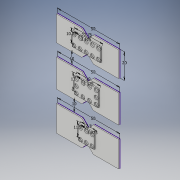
# Autodesk Inventor part: Templates
Saved by Autodesk Inventor 2017 (Build 210142000, 142)
## iProperties
Created: 2023-07-15
Part Number: Templates
Material: Generic
Document SubType Name: Modeling
Designer: Win240
Density: 1 g/cm^3
Appearance: Default
Author: Win240
Autodesk Inventor part; units mm, degrees
ref_plane "YZ Plane" through (0, 0, 0) normal (1, 0, 0) x (0, 1, 0)
ref_plane "XZ Plane" through (0, 0, 0) normal (0, 1, 0) x (-1, 0, 0)
ref_plane "XY Plane" through (0, 0, 0) normal (0, 0, 1) x (1, 0, 0)
sketch "Sketch1" plane through (0, 0, 0) normal (0, 0, 1) x (1, 0, 0)
  line L0 (-25, -11.125) -> (-4.625, -11.125)
  line L1 (25, -11.125) -> (25, 11.125)
  line L2 (25, 11.125) -> (4.625, 11.125)
  line L3 (-25, 11.125) -> (-25, -11.125)
  line L4 (-25, -11.125) -> (25, 11.125) construction
  line L5 (25, -11.125) -> (-25, 11.125) construction
  line L6 (-9.5, -6.5) -> (9.5, -6.5)
  line L7 (9.5, -6.5) -> (9.5, 6.5)
  line L8 (9.5, 6.5) -> (-9.5, 6.5)
  line L9 (-9.5, 6.5) -> (-9.5, -6.5)
  line L10 (-9.5, -6.5) -> (9.5, 6.5) construction
  line L11 (9.5, -6.5) -> (-9.5, 6.5) construction
  line L12 (0, 6.5) -> (-4.625, 11.125)
  line L13 (0, 6.5) -> (4.625, 11.125)
  line L14 (0, -6.5) -> (-4.625, -11.125)
  line L15 (0, -6.5) -> (4.625, -11.125)
  line L16 (-4.625, 11.125) -> (-25, 11.125)
  line L17 (4.625, -11.125) -> (25, -11.125)
  circle A0 centre (-7.9125, 4.9125) radius 1.5875
  circle A1 centre (-7.9125, -4.9125) radius 1.5875
  circle A2 centre (7.9125, -4.9125) radius 1.5875
  circle A3 centre (7.9125, 4.9125) radius 1.5875
  circle A4 centre (-2.6375, -4.9125) radius 1.5875
  circle A5 centre (2.6375, -4.9125) radius 1.5875
  circle A6 centre (2.6375, 4.9125) radius 1.5875
  circle A7 centre (-2.6375, 4.9125) radius 1.5875
  line L18 (-7.9125, 4.9125) -> (-2.6375, 4.9125) construction
  line L19 (2.6375, -4.9125) -> (2.6375, 4.9125) construction
  line L20 (-2.6375, 4.9125) -> (-2.6375, -4.9125) construction
  line L21 (-25, -41.675) -> (-4.625, -41.675)
  line L22 (25, -41.675) -> (25, -21.125)
  line L23 (25, -21.125) -> (4.625, -21.125)
  line L24 (-25, -21.125) -> (-25, -41.675)
  line L25 (-25, -41.675) -> (25, -21.125) construction
  line L26 (25, -41.675) -> (-25, -21.125) construction
  line L27 (-6.25, -37.05) -> (6.25, -37.05)
  line L28 (6.25, -37.05) -> (6.25, -25.75)
  line L29 (6.25, -25.75) -> (-6.25, -25.75)
  line L30 (-6.25, -25.75) -> (-6.25, -37.05)
  line L31 (-6.25, -37.05) -> (6.25, -25.75) construction
  line L32 (6.25, -37.05) -> (-6.25, -25.75) construction
  line L33 (0, -25.75) -> (-4.625, -21.125)
  line L34 (0, -25.75) -> (4.625, -21.125)
  line L35 (0, -37.05) -> (-4.625, -41.675)
  line L36 (0, -37.05) -> (4.625, -41.675)
  line L37 (-4.625, -21.125) -> (-25, -21.125)
  line L38 (4.625, -41.675) -> (25, -41.675)
  circle A8 centre (-4.6625, -27.3375) radius 1.5875
  circle A9 centre (-4.6625, -35.4625) radius 1.5875
  circle A10 centre (4.6625, -35.4625) radius 1.5875
  circle A11 centre (4.6625, -27.3375) radius 1.5875
  circle A12 centre (0, -27.3375) radius 1.5875
  circle A13 centre (0, -35.4625) radius 1.5875
  line L39 (-25, 21.125) -> (-4.625, 21.125)
  line L40 (25, 21.125) -> (25, 41.125)
  line L41 (25, 41.125) -> (4.625, 41.125)
  line L42 (-25, 41.125) -> (-25, 21.125)
  line L43 (-25, 21.125) -> (25, 41.125) construction
  line L44 (25, 21.125) -> (-25, 41.125) construction
  line L45 (-11.375, 25.75) -> (11.375, 25.75)
  line L46 (11.375, 25.75) -> (11.375, 36.5)
  line L47 (11.375, 36.5) -> (-11.375, 36.5)
  line L48 (-11.375, 36.5) -> (-11.375, 25.75)
  line L49 (-11.375, 25.75) -> (11.375, 36.5) construction
  line L50 (11.375, 25.75) -> (-11.375, 36.5) construction
  line L51 (0, 36.5) -> (-4.625, 41.125)
  line L52 (0, 36.5) -> (4.625, 41.125)
  line L53 (0, 25.75) -> (-4.625, 21.125)
  line L54 (0, 25.75) -> (4.625, 21.125)
  line L55 (-4.625, 41.125) -> (-25, 41.125)
  line L56 (4.625, 21.125) -> (25, 21.125)
  circle A14 centre (-9.7875, 34.9125) radius 1.5875
  circle A15 centre (-9.7875, 27.3375) radius 1.5875
  circle A16 centre (9.7875, 27.3375) radius 1.5875
  circle A17 centre (9.7875, 34.9125) radius 1.5875
  circle A18 centre (0, 34.9125) radius 1.5875
  circle A19 centre (0, 27.3375) radius 1.5875
  circle A20 centre (-4.8937, 27.3375) radius 1.5875
  circle A21 centre (4.8938, 27.3375) radius 1.5875
  circle A22 centre (4.8938, 34.9125) radius 1.5875
  circle A23 centre (-4.8937, 34.9125) radius 1.5875
  line L57 (-9.7875, 34.9125) -> (-4.8937, 34.9125) construction
  line L58 (-4.8937, 34.9125) -> (0, 34.9125) construction
  line L59 (0, 34.9125) -> (4.8938, 34.9125) construction
  line L60 (4.8938, 27.3375) -> (4.8938, 34.9125) construction
  line L61 (-4.8937, 34.9125) -> (-4.8937, 27.3375) construction
  line L62 (-2.6375, 4.9125) -> (2.6375, 4.9125) construction
  line L63 (2.6375, 4.9125) -> (7.9125, 4.9125) construction
  line L64 (9.5, 6.5) -> (9.5, 11.125) construction
  line L65 (11.375, 36.5) -> (11.375, 41.125) construction
  line L66 (6.25, -25.75) -> (6.25, -21.125) construction
  circle A24 centre (-7.9125, 0) radius 1.5875
  circle A25 centre (7.9125, 0) radius 1.5875
  point P0 (0, 0)
  point P1 (0, 0)
  point P2 (0, 0)
  point P3 (0, 0)
  point P4 (0, 0)
  point P5 (0, -31.4)
  point P6 (0, -31.4)
  point P7 (0, -31.4)
  point P8 (0, -31.4)
  point P9 (0, -31.4)
  point P10 (0, 31.125)
  point P11 (0, 31.125)
  point P12 (0, 31.125)
  point P13 (0, 31.125)
  point P14 (0, 31.125)
  dimension "d1" = 50
  dimension "d2" = 19
  dimension "d3" = 13
  dimension "d12" = 3.175
  dimension "d14" = 50
  dimension "d15" = 12.5
  dimension "d16" = 11.3
  dimension "d17" = 3.175
  dimension "d18" = 20
  dimension "d19" = 50
  dimension "d20" = 22.75
  dimension "d21" = 10.75
  dimension "d22" = 3.175
  dimension "d23" = 10
  dimension "d24" = 10
  constraints: 134 end point, 38 tangent, 30 midpoint, 26 centre point, 23 equal radius, 21 parallel, 15 perpendicular, 12 equal length, 9 horizontal, 7 vertical, 6 point on line, 6 vertical alignment, 3 collinear, 2 horizontal alignment
  measures "d1" distance of L1.end L3.start
  measures "d2" distance of L7.end L8.end
  measures "d3" distance of L8.end L6.start
  measures "d12" diameter of A0
  measures "d14" distance of L22.end L37.end
  measures "d15" distance of L31.end L30.start
  measures "d16" distance of L30.start L30.end
  measures "d17" diameter of A8
  measures "d18" distance of L44.start L43.end
  measures "d19" distance of L43.end L44.end
  measures "d20" distance of L46.end L48.start
  measures "d21" distance of L48.start L48.end
  measures "d22" diameter of A14
  measures "d23" distance between parallel lines of L39 L16
  measures "d24" distance between parallel lines of L0 L37
extrude "Extrusion1" add sketch "Sketch1" along normal blind 1 contours L3 L16 L12 L8 L9 L6 L14 L0 | A5 | A25 | A6 | A7 | A24 | A4 | L6 L7 L8 L13 L2 L1 L17 L15 | A1 | A2 | A3 | A0 | L24 L37 L33 L29 L30 L27 L35 L21 | A12 | L27 L28 L29 L34 L23 L22 L38 L36 | A13 | A9 | A10 | A11 | A8 | L42 L55 L51 L47 L48 L45 L53 L39 | A21 | A22 | A18 | A23 | A20 | L45 L46 L47 L52 L41 L40 L56 L54 | A19 | A15 | A16 | A17 | A14
extrude "Extrusion2" add sketch "Sketch1" along normal blind 2 contours L6 A1 L9 A0 L8 A3 L7 A2 | L6 L9 A1 | A2 L7 L6 | L8 L7 A3 | A0 L9 L8 | L27 A9 L30 A8 L29 A11 L28 A10 | L27 L30 A9 | A10 L28 L27 | L29 L28 A11 | A8 L30 L29 | L45 A15 L48 A14 L47 A17 L46 A16 | L45 L48 A15 | A16 L46 L45 | L47 L46 A17 | A14 L48 L47
body "Solid1"
